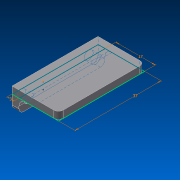
# Autodesk Inventor part: psu side brace
Saved by Autodesk Inventor 2015 (Build 190159000, 159)
## iProperties
Created: 2017-03-20
Part Number: psu side brace
Material: Generic
Document SubType Name: Modeling
Designer: ZigZagJoe
Density: 1 g/cm^3
Appearance: Default
Author: ZigZagJoe
Autodesk Inventor part; units mm, degrees
ref_plane "YZ Plane" through (0, 0, 0) normal (1, 0, 0) x (0, 1, 0)
ref_plane "XZ Plane" through (0, 0, 0) normal (0, 1, 0) x (-1, 0, 0)
ref_plane "XY Plane" through (0, 0, 0) normal (0, 0, 1) x (1, 0, 0)
sketch "Sketch1" plane through (0, 0, 0) normal (0, 0, 1) x (1, 0, 0)
  line L0 (-5.0801, 28.6808) -> (14.9199, 28.6808)
  line L1 (14.9199, 28.6808) -> (14.9199, -8.3192)
  line L2 (14.9199, -8.3192) -> (-5.0801, -8.3192)
  line L3 (-5.0801, -8.3192) -> (-5.0801, 28.6808)
  line L4 (-5.0801, 28.6808) -> (-2.0801, 28.6808)
  line L5 (-2.0801, 28.6808) -> (-2.0801, -8.3192)
  line L6 (-2.0801, -8.3192) -> (-5.0801, -8.3192)
  line L7 (-5.0801, -8.3192) -> (-5.0801, 28.6808)
  point P0 (0, 0)
  dimension "d0" = 3
  dimension "d1" = 17
  dimension "d12" = 37
  constraints: 16 end point, 4 parallel, 2 horizontal, 2 perpendicular, 1 point on line
  measures "d0" distance of L5.end L6.end
  measures "d1" distance between parallel lines of L1 L5
  measures "d12" distance of L0.end L1.end
extrude "Extrusion1" add sketch "Sketch1" along normal blind 3
extrude "Extrusion2" add sketch "Sketch1" against normal blind 6 contours L0 L5 L2 L3
sketch "Sketch2" plane through (-5.0801, -8.3192, 3) normal (-1, 0, 0) x (0, 0, 1)
  circle A0 centre (-5, 4) radius 1.9
  circle A1 centre (-5, 33) radius 1.9
  line L0 (-3, 0) -> (-3, 37) projected
  line L1 (-9, 0) -> (0, 0) projected
  line L2 (-9, 37) -> (0, 37) projected
  line L3 (-9, 0) -> (-9, 37) projected
  line L4 (0, 37) -> (0, 0) projected
  point P0 (-3, 8.3192)
  dimension "d6" = 3.8
  dimension "d7" = 3.8
  dimension "d10" = 4
  dimension "d11" = 4
  dimension "d17" = 4
  dimension "d18" = 4
  dimension "d19" = 5
  constraints: 2 centre point
  measures "d6" diameter of A0
  measures "d7" diameter of A1
  measures "d10" distance from line of L1 A0.centre
  measures "d11" distance from line of L2 A1.centre
  measures "d17" distance from line of L3 A1.centre
  measures "d18" distance from line of L3 A0.centre
  measures "d19" distance from line of L4 A0.centre
extrude "Extrusion3" cut sketch "Sketch2" against normal blind 6 contours A0 | A1
fillet "Fillet1" radius 3 1 edges at (-2.0801, 10.1808, 0)
fillet "Fillet2" radius 2 4 edges at (-3.5801, 28.6808, -6) (-3.5801, -8.3192, -6) (14.9199, 28.6808, 1.5) (14.9199, -8.3192, 1.5)
sketch "Sketch3" plane through (0, 0, 3) normal (0, 0, 1) x (1, 0, 0)
  point P0 (0, 0)
body "Solid1"
